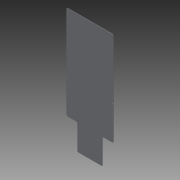
# Autodesk Inventor part: Back plate
Saved by Autodesk Inventor 2015 (Build 190159000, 159)
## iProperties
Created: 2015-01-17
Part Number: Back plate
Material: Generic
Document SubType Name: Modeling
Designer: chapale16
Density: 1 g/cm^3
Appearance: Default
Author: chapale16
Autodesk Inventor part; units mm, degrees
ref_plane "YZ Plane" through (0, 0, 0) normal (1, 0, 0) x (0, 1, 0)
ref_plane "XZ Plane" through (0, 0, 0) normal (0, 1, 0) x (-1, 0, 0)
ref_plane "XY Plane" through (0, 0, 0) normal (0, 0, 1) x (1, 0, 0)
sketch "Sketch2" plane through (0, 0, 0) normal (0, 0, 1) x (1, 0, 0)
  line L0 (0, 0) -> (566.42, 0)
  line L1 (566.42, 0) -> (566.42, -1727.2)
  line L2 (566.42, -1727.2) -> (0, -1727.2)
  line L3 (0, -1727.2) -> (0, 0)
  dimension "d0" = 566.42
  dimension "d1" = 1727.2
  constraints: 8 end point, 2 parallel, 1 horizontal, 1 perpendicular
  measures "d0" distance of L1.end L2.end
  measures "d1" distance of L0.end L1.end
extrude "Extrusion1" add sketch "Sketch2" along normal blind 3.175
sketch "Sketch4" plane through (0, 0, 3.175) normal (0, 0, 1) x (1, 0, 0)
  line L0 (566.42, 0) -> (0, 0) projected
  line L1 (0, 0) -> (0, -1727.2) projected
  line L2 (0, -1727.2) -> (566.42, -1727.2) projected
  line L3 (566.42, -1727.2) -> (566.42, 0) projected
  line L4 (0, -1727.2) -> (566.42, -1727.2) projected
  line L5 (68.58, -1727.2) -> (500.38, -1727.2)
  circle A0 centre (68.58, -1391.92) radius 12.7
  circle A1 centre (500.38, -1391.92) radius 12.7
  circle A2 centre (68.58, -1727.2) radius 12.7
  circle A3 centre (500.38, -1727.2) radius 12.7
  dimension "d6" = 25.4
  dimension "d7" = 25.4
  dimension "d8" = 25.4
  dimension "d9" = 25.4
  constraints: 4 centre point, 2 coincident, 2 end point, 1 horizontal, 1 point on line
  measures "d6" diameter of A0
  measures "d7" diameter of A1
  measures "d8" diameter of A2
  measures "d9" diameter of A3
extrude "Extrusion2" add sketch "Sketch4" along normal blind 3.175 contours A0 | A1
sketch "Sketch6" plane through (0, 0, 3.175) normal (0, 0, 1) x (1, 0, 0)
  circle A0 centre (12.7, -1460.5) radius 3.175 projected
  circle A1 centre (553.72, -1460.5) radius 3.175 projected
  circle A2 centre (553.72, -1460.5) radius 4.7625
  circle A3 centre (12.7, -1460.5) radius 4.7625
  point P0 (0, 0)
  dimension "d16" = 9.525
  dimension "d17" = 9.525
  constraints: 2 centre point, 2 coincident
  measures "d16" diameter of A2
  measures "d17" diameter of A3
extrude "Extrusion4" cut sketch "Sketch6" against normal through all contours A0 | A1 | A2 | A3
sketch "Sketch7" plane through (0, 0, 3.175) normal (0, 0, 1) x (1, 0, 0)
  circle A0 centre (12.7, -1460.5) radius 4.7625 projected
  circle A1 centre (12.7, -1460.5) radius 6.35
  circle A2 centre (553.72, -1460.5) radius 4.7625 projected
  circle A3 centre (553.72, -1460.5) radius 6.35
  point P0 (0, 0)
  dimension "d20" = 12.7
  dimension "d21" = 12.7
  constraints: 2 centre point, 2 coincident
  measures "d20" diameter of A1
  measures "d21" diameter of A3
extrude "Extrusion5" cut sketch "Sketch7" against normal blind 12.7 contours A3
sketch "Sketch9" plane through (0, 0, 3.175) normal (0, 0, 1) x (1, 0, 0)
  circle A0 centre (553.72, -825.5) radius 6.35 projected
  circle A1 centre (12.7, -825.5) radius 6.35 projected
  circle A2 centre (12.7, -825.5) radius 6.35
  circle A3 centre (553.72, -825.5) radius 6.35
  point P0 (0, 0)
  constraints: 2 centre point, 2 coincident, 2 concentric
extrude "Extrusion7" cut sketch "Sketch9" against normal blind 3.175
sketch "Sketch10" plane through (0, 0, 3.175) normal (0, 0, 1) x (1, 0, 0)
  line L0 (566.42, 0) -> (566.42, -1727.2) projected
  line L1 (0, -1732.8892) -> (566.42, -1732.8892)
  line L2 (566.42, -1732.8892) -> (566.42, -1054.0894)
  line L3 (566.42, -1054.0894) -> (0, -1054.0894)
  line L4 (0, -1054.0894) -> (0, -1732.8892)
  point P0 (0, 0)
  constraints: 8 end point, 2 parallel, 1 horizontal, 1 perpendicular, 1 point on line
extrude "Extrusion8" cut sketch "Sketch10" along normal blind 25.4
sketch "Sketch12" plane through (0, 0, 0) normal (0, 0, -1) x (-1, 0, 0)
  line L0 (-133.5248, -1752.8599) -> (-130.3498, -1752.8599) projected
  line L1 (-130.3498, -1752.8599) -> (-130.3498, -1726.7719) projected
  line L2 (-130.3498, -1726.7719) -> (-133.5248, -1726.7719) projected
  line L3 (-133.5248, -1726.7719) -> (-133.5248, -1752.8599) projected
  line L4 (-133.5248, -1752.8599) -> (-130.3498, -1752.8599) projected
  line L5 (-133.5248, -1777.5719) -> (-133.5248, -1752.8599) projected
  line L6 (-82.7248, -1777.5719) -> (-133.5248, -1777.5719) projected
  line L7 (-82.7248, -1774.3969) -> (-82.7248, -1777.5719) projected
  line L8 (-130.3498, -1774.3969) -> (-82.7248, -1774.3969) projected
  line L9 (-130.3498, -1752.8599) -> (-130.3498, -1774.3969) projected
  line L10 (-130.3498, -1237.6912) -> (0, -1237.6912)
  line L11 (0, -1237.6912) -> (0, -1727.2)
  line L12 (0, -1727.2) -> (-130.3498, -1727.2)
  line L13 (-130.3498, -1727.2) -> (-130.3498, -1237.6912)
  line L14 (0, -1727.2) -> (-566.42, -1727.2) projected
  line L15 (-566.8989, -1237.6912) -> (-436.5461, -1237.6912)
  line L16 (-436.5461, -1237.6912) -> (-436.5461, -1727.2)
  line L17 (-436.5461, -1727.2) -> (-566.8989, -1727.2)
  line L18 (-566.8989, -1727.2) -> (-566.8989, -1237.6912)
  point P0 (0, 0)
  point P1 (-108.1248, -1263.0912)
  dimension "d32" = 130.3528
  constraints: 16 end point, 4 parallel, 2 horizontal, 2 perpendicular, 2 point on line
  measures "d32" distance of L16.end L17.end
extrude "Extrusion9" cut sketch "Sketch12" against normal blind 3.175 contours L1 L13 L10 L11 L12
sketch "Sketch13" plane through (0, 0, 0) normal (0, 0, -1) x (-1, 0, 0)
  line L0 (-566.42, -1727.2) -> (-566.42, 0) projected
  line L1 (-130.3498, -1727.2) -> (-566.42, -1727.2) projected
  line L2 (-566.42, -1239.5747) -> (-435.131, -1239.5747)
  line L3 (-435.131, -1239.5747) -> (-435.131, -1727.2)
  line L4 (-435.131, -1727.2) -> (-566.42, -1727.2)
  line L5 (-566.42, -1727.2) -> (-566.42, -1239.5747)
  point P0 (0, 0)
  constraints: 8 end point, 2 parallel, 2 point on line, 1 horizontal, 1 perpendicular
extrude "Extrusion10" cut sketch "Sketch13" against normal blind 3.175
sketch "Sketch14" plane through (0, 0, 0) normal (0, 0, -1) x (-1, 0, 0)
  line L0 (-130.3498, -1727.2) -> (-130.3498, -1237.6912) projected
  line L1 (-435.131, -1727.2) -> (-130.3498, -1727.2)
  line L2 (-130.3498, -1727.2) -> (-130.3498, -1549.4)
  line L3 (-130.3498, -1549.4) -> (-435.131, -1549.4)
  line L4 (-435.131, -1549.4) -> (-435.131, -1727.2)
  point P0 (0, 0)
  dimension "d35" = 177.8
  constraints: 8 end point, 2 parallel, 1 horizontal, 1 perpendicular, 1 point on line
  measures "d35" distance of L2.end L1.end
extrude "Extrusion11" cut sketch "Sketch14" against normal blind 3.175
hole "Hole1" at (12.7, -12.7, 3.175) direction (0, 0, -1) diameter 6.35 depth 12.7 tip angle 118
pattern_linear "Rectangular Pattern1" count 17 spacing 76.2 along (0, -1, 0) of "Hole1"
hole "Hole2" at (553.72, -12.7, 3.175) direction (0, 0, -1) diameter 6.35 depth 12.7 tip angle 118
pattern_linear "Rectangular Pattern2" count 17 spacing 76.2 along (0, -1, 0) of "Hole2"
fillet "Fillet1" radius 12.7 8 edges at (566.42, 0, 1.5875) (0, 0, 1.5875) (566.42, -1239.5747, 1.5875) (435.131, -1239.5747, 1.5875) (435.131, -1549.4, 1.5875) (0, -1237.6912, 1.5875) (130.3498, -1237.6912, 1.5875) (130.3498, -1549.4, 1.5875)
sketch "Sketch15" plane through (0, 0, 3.175) normal (0, 0, 1) x (1, 0, 0)
  arc A0 (130.3498, -1536.7) -> (143.0498, -1549.4) centre (143.0498, -1536.7) ccw projected
  line L0 (143.0498, -1549.4) -> (422.431, -1549.4) projected
  arc A1 (422.431, -1549.4) -> (435.131, -1536.7) centre (422.431, -1536.7) ccw projected
  line L1 (435.131, -1536.7) -> (435.131, -1252.2747) projected
  arc A2 (447.831, -1239.5747) -> (435.131, -1252.2747) centre (447.831, -1252.2747) ccw projected
  line L2 (447.831, -1239.5747) -> (553.72, -1239.5747) projected
  arc A3 (553.72, -1239.5747) -> (566.42, -1226.8747) centre (553.72, -1226.8747) ccw projected
  line L3 (566.42, -1226.8747) -> (566.42, -12.7) projected
  arc A4 (566.42, -12.7) -> (553.72, 0) centre (553.72, -12.7) ccw projected
  line L4 (553.72, 0) -> (12.7, 0) projected
  arc A5 (12.7, 0) -> (0, -12.7) centre (12.7, -12.7) ccw projected
  line L5 (0, -12.7) -> (0, -1224.9912) projected
  arc A6 (0, -1224.9912) -> (12.7, -1237.6912) centre (12.7, -1224.9912) ccw projected
  line L6 (12.7, -1237.6912) -> (117.6498, -1237.6912) projected
  arc A7 (130.3498, -1250.3912) -> (117.6498, -1237.6912) centre (117.6498, -1250.3912) ccw projected
  line L7 (130.3498, -1250.3912) -> (130.3498, -1536.7) projected
  circle A8 centre (12.7, -825.5) radius 6.35 projected
  circle A9 centre (553.72, -825.5) radius 6.35 projected
  circle A10 centre (12.7, -12.7) radius 3.175 projected
  circle A11 centre (12.7, -88.9) radius 3.175 projected
  circle A12 centre (12.7, -165.1) radius 3.175 projected
  circle A13 centre (12.7, -241.3) radius 3.175 projected
  circle A14 centre (12.7, -317.5) radius 3.175 projected
  circle A15 centre (12.7, -393.7) radius 3.175 projected
  circle A16 centre (12.7, -469.9) radius 3.175 projected
  circle A17 centre (12.7, -546.1) radius 3.175 projected
  circle A18 centre (12.7, -622.3) radius 3.175 projected
  circle A19 centre (12.7, -698.5) radius 3.175 projected
  circle A20 centre (12.7, -774.7) radius 3.175 projected
  circle A21 centre (12.7, -850.9) radius 3.175 projected
  circle A22 centre (12.7, -927.1) radius 3.175 projected
  circle A23 centre (12.7, -1003.3) radius 3.175 projected
  circle A24 centre (12.7, -1079.5) radius 3.175 projected
  circle A25 centre (12.7, -1155.7) radius 3.175 projected
  circle A26 centre (12.7, -1231.9) radius 3.175 projected
  circle A27 centre (553.72, -12.7) radius 3.175 projected
  circle A28 centre (553.72, -88.9) radius 3.175 projected
  circle A29 centre (553.72, -165.1) radius 3.175 projected
  circle A30 centre (553.72, -241.3) radius 3.175 projected
  circle A31 centre (553.72, -317.5) radius 3.175 projected
  circle A32 centre (553.72, -393.7) radius 3.175 projected
  circle A33 centre (553.72, -469.9) radius 3.175 projected
  circle A34 centre (553.72, -546.1) radius 3.175 projected
  circle A35 centre (553.72, -622.3) radius 3.175 projected
  circle A36 centre (553.72, -698.5) radius 3.175 projected
  circle A37 centre (553.72, -774.7) radius 3.175 projected
  circle A38 centre (553.72, -850.9) radius 3.175 projected
  circle A39 centre (553.72, -927.1) radius 3.175 projected
  circle A40 centre (553.72, -1003.3) radius 3.175 projected
  circle A41 centre (553.72, -1079.5) radius 3.175 projected
  circle A42 centre (553.72, -1155.7) radius 3.175 projected
  circle A43 centre (553.72, -1231.9) radius 3.175 projected
  line L8 (0, 0) -> (566.42, 0)
  line L9 (566.42, 0) -> (566.42, -101.6)
  line L10 (566.42, -101.6) -> (0, -101.6)
  line L11 (0, -101.6) -> (0, 0)
  dimension "d63" = 101.6
  constraints: 8 end point, 2 parallel, 1 horizontal, 1 perpendicular, 1 point on line
  measures "d63" distance of L8.end L9.end
extrude "Extrusion12" cut sketch "Sketch15" against normal blind 25.4 contours L5 A5 L4 A4 L3 L10 | L11 L8 A5 | A4 L8 L9
fillet "Fillet2" radius 12.7 1 edges at (566.42, -101.6, 1.5875)
fillet "Fillet3" radius 12.7 1 edges at (0, -101.6, 1.5875)
equation "\"d22\" = d20"
body "Solid1"
